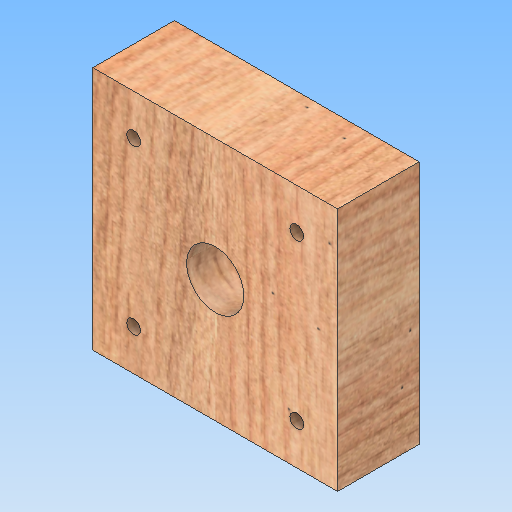
# Autodesk Inventor part: Top_Spacer
Saved by Autodesk Inventor 2018.1 (Build 221171000, 171)
## iProperties
Created: 2019-03-15
Part Number: Top_Spacer
Material: Wood (Birch)
Document SubType Name: Modeling
Designer: James
Density: 0.55 g/cm^3
Appearance: Birch - Natural Polished
Mass: 585.501 g
Surface Area: 832.676 cm^2
Volume: 1064.55 cm^3
Author: James
Autodesk Inventor part; units mm, degrees
ref_plane "YZ Plane" through (0, 0, 0) normal (1, 0, 0) x (0, 1, 0)
ref_plane "XZ Plane" through (0, 0, 0) normal (0, 1, 0) x (-1, 0, 0)
ref_plane "XY Plane" through (0, 0, 0) normal (0, 0, 1) x (1, 0, 0)
sketch "Sketch1" plane through (0, 0, 0) normal (0, 0, 1) x (1, 0, 0)
  line L0 (0, 0) -> (150, 0)
  line L1 (150, 0) -> (150, 150)
  line L2 (150, 150) -> (0, 150)
  line L3 (0, 150) -> (0, 0)
  dimension "d0" = 150
  dimension "d1" = 150
  constraints: 8 end point, 2 parallel, 1 horizontal, 1 perpendicular
  measures "d0" distance of L2.end L1.end
  measures "d1" distance of L1.end L0.end
extrude "Extrusion1" add sketch "Sketch1" along normal blind 50
sketch "Sketch2" plane through (0, 0, 50) normal (0, 0, 1) x (1, 0, 0)
  line L0 (150, 0) -> (150, 150) projected
  line L1 (150, 150) -> (0, 150) projected
  point P0 (0, 0)
  point P1 (75, 75)
  point P2 (150, 75)
  point P3 (75, 150)
  constraints: 2 midpoint, 1 horizontal alignment, 1 vertical alignment
hole "Hole1" at (75, 75, 50) direction (0, 0, -1) diameter 35 end through all
sketch "Sketch3" plane through (0, 0, 0) normal (0, 0, -1) x (-1, 0, 0)
  line L0 (-150, 150) -> (0, 150) projected
  line L1 (0, 150) -> (0, 0) projected
  line L2 (0, 0) -> (-150, 0) projected
  line L3 (-150, 0) -> (-150, 150) projected
  point P0 (-125, 125)
  point P1 (-25, 125)
  point P2 (-25, 25)
  point P3 (-125, 25)
  dimension "d11" = 25
  dimension "d12" = 25
  dimension "d13" = 25
  dimension "d14" = 25
  constraints: 2 horizontal alignment, 2 vertical alignment
  measures "d11" distance from line of L0 point (-125, 125)
  measures "d12" distance from line of L1 point (-25, 125)
  measures "d13" distance from line of L2 point (-125, 25)
  measures "d14" distance from line of L3 point (-125, 125)
hole "Hole2" at (125, 125, 0) at (25, 125, 0) at (25, 25, 0) at (125, 25, 0) direction (0, 0, 1) diameter 8.433 end through all countersink diameter 16.129 countersink angle 82 clearance for "Flat Head Machine Screw (82)" size "5/16" standard "Ansi Unified Screw Threads"
equation "\"d12\" = d11"
equation "\"d13\" = d11"
equation "\"d14\" = d11"
body "Solid1"
